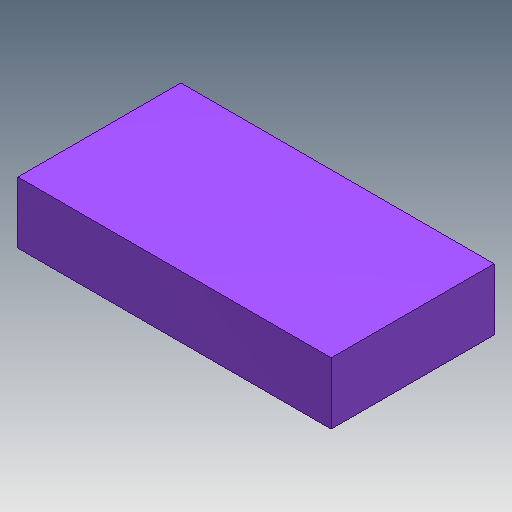
# Autodesk Inventor part: EXTERNAL
Saved by Autodesk Inventor 2017 (Build 210142000, 142)
## iProperties
Part Number: EXTERNAL
Material: Generisch
Document SubType Name: Modeling
Designer: Werkstatt
Density: 1 g/cm^3
Appearance: 1X02, EXTERNAL
Author: Werkstatt
Autodesk Inventor part; units mm, degrees
ref_plane "YZ Plane" through (0, 0, 0) normal (1, 0, 0) x (0, 1, 0)
ref_plane "XZ Plane" through (0, 0, 0) normal (0, 1, 0) x (-1, 0, 0)
ref_plane "XY Plane" through (0, 0, 0) normal (0, 0, 1) x (1, 0, 0)
sketch "1X02, EXTERNAL_32" plane through (0, 0, 0) normal (0, 0, 1) x (1, 0, 0)
  line L0 (-1.27, 1.3716) -> (3.81, 1.3716)
  line L1 (3.81, 1.3716) -> (3.81, -1.27)
  line L2 (3.81, -1.27) -> (-1.27, -1.27)
  line L3 (-1.27, -1.27) -> (-1.27, 1.3716)
  constraints: 8 end point
extrude "Extrusion1" add sketch "1X02, EXTERNAL_32" along normal blind 1
